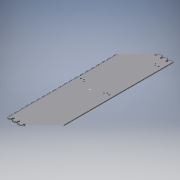
# Autodesk Inventor part: 3DPrinterBracket_bottom
Saved by Autodesk Inventor 2016 (Build 200138000, 138)
## iProperties
Created: 2017-10-03
Part Number: 3DPrinterBracket_bottom
Material: Generic
Document SubType Name: Modeling
Designer: jcj2131
Density: 1 g/cm^3
Appearance: Default
Author: jcj2131
Autodesk Inventor part; units mm, degrees
ref_plane "YZ Plane" through (0, 0, 0) normal (1, 0, 0) x (0, 1, 0)
ref_plane "XZ Plane" through (0, 0, 0) normal (0, 1, 0) x (-1, 0, 0)
ref_plane "XY Plane" through (0, 0, 0) normal (0, 0, 1) x (1, 0, 0)
sketch "Sketch1" plane through (0, 0, 0) normal (0, 1, 0) x (-1, 0, 0)
  line L0 (82.55, 306.3875) -> (-82.55, 306.3875)
  line L1 (-82.55, 306.3875) -> (-82.55, -306.3875)
  line L2 (-82.55, -306.3875) -> (82.55, -306.3875)
  line L3 (82.55, -306.3875) -> (82.55, 306.3875)
  point P0 (0, 0)
  point P1 (0, 306.3875)
  point P2 (82.55, 0)
  dimension "d0" = 612.775
  dimension "d1" = 165.1
  constraints: 8 end point, 2 midpoint, 2 parallel, 1 horizontal, 1 horizontal alignment, 1 perpendicular, 1 vertical alignment
  measures "d0" distance of L2.end L0.start
  measures "d1" distance of L0.start L0.end
extrude "Extrusion1" add sketch "Sketch1" along normal blind 3.175
sketch "Sketch2" plane through (0, 3.175, 0) normal (0, 1, 0) x (1, 0, 0)
  line L0 (-82.55, -306.3875) -> (82.55, -306.3875) projected
  line L1 (-69.85, -306.3875) -> (-57.15, -306.3875)
  line L2 (-57.15, -306.3875) -> (-57.15, -303.2125)
  line L3 (-57.15, -303.2125) -> (-69.85, -303.2125)
  line L4 (-69.85, -303.2125) -> (-69.85, -306.3875)
  line L5 (-82.55, 306.3875) -> (-82.55, -306.3875) projected
  point P0 (0, 0)
  dimension "d4" = 12.7
  dimension "d5" = 12.7
  dimension "d6" = 3.175
  constraints: 8 end point, 2 parallel, 1 horizontal, 1 perpendicular, 1 point on line
  measures "d4" distance between parallel lines of L5 L4
  measures "d5" distance of L2.end L3.end
  measures "d6" distance of L1.end L2.end
extrude "Extrusion2" cut sketch "Sketch2" against normal through all
sketch "Sketch3" plane through (0, 3.175, 0) normal (0, 1, 0) x (1, 0, 0)
  line L0 (-57.15, -303.2125) -> (-69.85, -303.2125) projected
  line L1 (-65.278, -303.2125) -> (-61.722, -303.2125)
  line L2 (-61.722, -303.2125) -> (-61.722, -297.2125)
  line L3 (-61.722, -297.2125) -> (-65.278, -297.2125)
  line L4 (-65.278, -297.2125) -> (-65.278, -303.2125)
  line L5 (-69.85, -306.3875) -> (-69.85, -303.2125) projected
  point P0 (0, 0)
  dimension "d9" = 3.556
  dimension "d10" = 6
  dimension "d11" = 4.572
  constraints: 8 end point, 2 parallel, 1 horizontal, 1 perpendicular, 1 point on line
  measures "d9" distance of L2.end L3.end
  measures "d10" distance of L3.end L1.start
  measures "d11" distance between parallel lines of L5 L4
extrude "Extrusion3" cut sketch "Sketch3" against normal through all
sketch "Sketch4" plane through (0, 3.175, 0) normal (0, 1, 0) x (1, 0, 0)
  line L0 (-59.5315, -297.2125) -> (-67.469, -297.2125)
  line L1 (-67.469, -297.2125) -> (-67.469, -294.4345)
  line L2 (-67.469, -294.4345) -> (-59.5315, -294.4345)
  line L3 (-59.5315, -294.4345) -> (-59.5315, -297.2125)
  line L4 (-65.278, -297.2125) -> (-61.722, -297.2125) projected
  line L5 (-69.85, -306.3875) -> (-69.85, -303.2125) projected
  point P0 (0, 0)
  dimension "d14" = 7.9375
  dimension "d15" = 2.778
  dimension "d16" = 0
  dimension "d17" = 2.381
  constraints: 8 end point, 2 parallel, 1 horizontal, 1 perpendicular
  measures "d14" distance of L1.end L2.end
  measures "d15" distance of L0.end L1.end
  measures "d16" distance between parallel lines of L4 L0
  measures "d17" distance between parallel lines of L5 L1
extrude "Extrusion4" cut sketch "Sketch4" against normal through all
sketch "Sketch5" plane through (0, 3.175, 0) normal (0, 1, 0) x (1, 0, 0)
  line L0 (-59.5315, -294.4345) -> (-67.469, -294.4345) projected
  line L1 (-65.278, -294.4345) -> (-61.722, -294.4345)
  line L2 (-61.722, -294.4345) -> (-61.722, -291.1475)
  line L3 (-61.722, -291.1475) -> (-65.278, -291.1475)
  line L4 (-65.278, -291.1475) -> (-65.278, -294.4345)
  line L5 (-69.85, -306.3875) -> (-69.85, -303.2125) projected
  line L6 (-57.15, -306.3875) -> (82.55, -306.3875) projected
  point P0 (0, 0)
  dimension "d20" = 3.556
  dimension "d21" = 4.572
  dimension "d22" = 15.24
  constraints: 8 end point, 2 parallel, 1 horizontal, 1 perpendicular, 1 point on line
  measures "d20" distance of L2.end L3.end
  measures "d21" distance between parallel lines of L5 L4
  measures "d22" distance between parallel lines of L6 L3
extrude "Extrusion5" cut sketch "Sketch5" against normal through all
pattern_linear "Rectangular Pattern1" count 6 spacing 25.4 along (1, 0, 0) of "Extrusion2", "Extrusion3", "Extrusion4", "Extrusion5"
sketch "Sketch6" plane through (0, 3.175, 0) normal (0, 1, 0) x (1, 0, 0)
  point P0 (0, 0)
mirror "Mirror1" about plane through (0, 0, 0) normal (0, 0, 1) of "Extrusion5", "Extrusion2", "Extrusion3", "Extrusion4", "Rectangular Pattern1"
sketch "Sketch7" plane through (0, 3.175, 0) normal (0, 1, 0) x (1, 0, 0)
  point P0 (0, 0)
sketch "Sketch8" plane through (0, 3.175, 0) normal (0, 1, 0) x (1, 0, 0)
  line L0 (-50.8, 22.3875) -> (50.8, 22.3875)
  line L1 (50.8, 22.3875) -> (50.8, 255.5875)
  line L2 (50.8, 255.5875) -> (-50.8, 255.5875)
  line L3 (-50.8, 255.5875) -> (-50.8, 22.3875)
  line L4 (-61.5, 148.8875) -> (61.5, 148.8875)
  line L5 (61.5, 148.8875) -> (61.5, 248.8875)
  line L6 (61.5, 248.8875) -> (-61.5, 248.8875)
  line L7 (-61.5, 248.8875) -> (-61.5, 148.8875)
  line L8 (82.55, -306.3875) -> (82.55, 306.3875) projected
  line L9 (-82.55, 306.3875) -> (-82.55, -306.3875) projected
  line L10 (-19.05, 306.3875) -> (-31.75, 306.3875) projected
  line L11 (-69.85, 306.3875) -> (-82.55, 306.3875) projected
  circle A0 centre (-57.5, 244.8875) radius 2.54
  circle A1 centre (-57.5, 152.8875) radius 2.54
  circle A2 centre (57.5, 152.8875) radius 2.54
  circle A3 centre (57.5, 244.8875) radius 2.54
  line L12 (-69.85, 306.3875) -> (-82.55, 306.3875) projected
  circle A4 centre (-54.61, 26.4875) radius 1.85
  circle A5 centre (-46.7, 18.5775) radius 1.85
  circle A6 centre (46.7, 18.5775) radius 1.85
  circle A7 centre (54.61, 26.4875) radius 1.85
  circle A8 centre (-54.61, 251.4875) radius 1.85
  circle A9 centre (-46.7, 259.3975) radius 1.85
  circle A10 centre (54.61, 251.4875) radius 1.85
  circle A11 centre (46.7, 259.3975) radius 1.85
  line L13 (-61.5, 128.8875) -> (61.5, 128.8875)
  line L14 (61.5, 128.8875) -> (61.5, 28.8875)
  line L15 (61.5, 28.8875) -> (-61.5, 28.8875)
  line L16 (-61.5, 28.8875) -> (-61.5, 128.8875)
  line L17 (-71.5, 258.8875) -> (-26.5, 258.8875)
  line L18 (-26.5, 258.8875) -> (-26.5, 18.8875)
  line L19 (-26.5, 18.8875) -> (-71.5, 18.8875)
  line L20 (-71.5, 18.8875) -> (-71.5, 258.8875)
  circle A12 centre (-66.5, 253.8875) radius 2.5
  circle A13 centre (-66.5, 23.8875) radius 2.5
  line L21 (26.5, 258.8875) -> (71.5, 258.8875)
  line L22 (71.5, 258.8875) -> (71.5, 18.8875)
  line L23 (71.5, 18.8875) -> (26.5, 18.8875)
  line L24 (26.5, 18.8875) -> (26.5, 258.8875)
  circle A14 centre (66.5, 253.8875) radius 2.5
  circle A15 centre (66.5, 23.8875) radius 2.5
  point P0 (0, 0)
  dimension "d28" = 233.2
  dimension "d29" = 101.6
  dimension "d30" = 100
  dimension "d31" = 123
  dimension "d36" = 5.08
  dimension "d37" = 4
  dimension "d38" = 4
  dimension "d39" = 5.08
  dimension "d40" = 4
  dimension "d41" = 4
  dimension "d42" = 5.08
  dimension "d43" = 4
  dimension "d44" = 4
  dimension "d45" = 5.08
  dimension "d46" = 4
  dimension "d47" = 4
  dimension "d73" = 21.05
  dimension "d74" = 10.7
  dimension "d75" = 50.8
  dimension "d76" = 57.5
  dimension "d77" = 3.7
  dimension "d78" = 3.81
  dimension "d79" = 4.1
  dimension "d80" = 3.7
  dimension "d81" = 3.81
  dimension "d82" = 4.1
  dimension "d83" = 3.7
  dimension "d84" = 3.81
  dimension "d85" = 4.1
  dimension "d86" = 3.7
  dimension "d87" = 3.81
  dimension "d88" = 3.7
  dimension "d89" = 3.81
  dimension "d90" = 4.1
  dimension "d91" = 3.7
  dimension "d92" = 3.81
  dimension "d93" = 4.1
  dimension "d94" = 3.7
  dimension "d95" = 3.81
  dimension "d96" = 4.1
  dimension "d97" = 3.7
  dimension "d98" = 3.81
  dimension "d99" = 4.1
  dimension "d109" = 4.1
  dimension "d118" = 20
  dimension "d119" = 240
  dimension "d120" = 45
  dimension "d121" = 14
  dimension "d122" = 14
  dimension "d123" = 5
  dimension "d124" = 5
  dimension "d125" = 5
  dimension "d126" = 5
  dimension "d127" = 5
  dimension "d128" = 5
  dimension "d129" = 53
  dimension "d130" = 5
  dimension "d131" = 5
  dimension "d132" = 5
  dimension "d133" = 14
  dimension "d134" = 5
  dimension "d135" = 5
  dimension "d136" = 5
  constraints: 40 end point, 16 centre point, 10 parallel, 5 horizontal, 5 perpendicular, 4 equal length
  measures "d28" distance of L2.end L0.start
  measures "d29" distance of L0.start L0.end
  measures "d30" distance of L6.end L4.start
  measures "d31" distance of L5.end L6.end
  measures "d36" diameter of A0
  measures "d37" distance from line of L6 A0.centre
  measures "d38" distance from line of L7 A0.centre
  measures "d39" diameter of A1
  measures "d40" distance from line of L7 A1.centre
  measures "d41" distance from line of L4 A1.centre
  measures "d42" diameter of A2
  measures "d43" distance from line of L5 A2.centre
  measures "d44" distance from line of L4 A2.centre
  measures "d45" diameter of A3
  measures "d46" distance from line of L5 A3.centre
  measures "d47" distance from line of L6 A3.centre
  measures "d73" distance between parallel lines of L8 L5
  measures "d74" distance between parallel lines of L5 L1
  measures "d75" distance between parallel lines of L11 L2
  measures "d76" distance between parallel lines of L12 L6
  measures "d77" diameter of A4
  measures "d78" distance from line of L3 A4.centre
  measures "d79" distance from line of L0 A4.centre
  measures "d80" diameter of A5
  measures "d81" distance from line of L0 A5.centre
  measures "d82" distance from line of L3 A5.centre
  measures "d83" diameter of A6
  measures "d84" distance from line of L0 A6.centre
  measures "d85" distance from line of L1 A6.centre
  measures "d86" diameter of A7
  measures "d87" distance from line of L1 A7.centre
  measures "d88" diameter of A8
  measures "d89" distance from line of L3 A8.centre
  measures "d90" distance from line of L2 A8.centre
  measures "d91" diameter of A9
  measures "d92" distance from line of L2 A9.centre
  measures "d93" distance from line of L3 A9.centre
  measures "d94" diameter of A10
  measures "d95" distance from line of L1 A10.centre
  measures "d96" distance from line of L2 A10.centre
  measures "d97" diameter of A11
  measures "d98" distance from line of L2 A11.centre
  measures "d99" distance from line of L1 A11.centre
  measures "d109" distance from line of L0 A7.centre
  measures "d118" distance between parallel lines of L13 L4
  measures "d119" distance of L19.end L17.start
  measures "d120" distance of L17.start L17.end
  measures "d121" distance from line of L20 A0.centre
  measures "d122" distance from line of A0.centre L17
  measures "d123" diameter of A12
  measures "d124" distance from line of L17 A12.centre
  measures "d125" distance from line of L20 A12.centre
  measures "d126" diameter of A13
  measures "d127" distance from line of L20 A13.centre
  measures "d128" distance from line of L19 A13.centre
  measures "d129" distance between parallel lines of L18 L24
  measures "d130" diameter of A14
  measures "d131" distance from line of L21 A14.centre
  measures "d132" distance from line of L22 A14.centre
  measures "d133" distance from line of L21 A3.centre
  measures "d134" diameter of A15
  measures "d135" distance from line of L22 A15.centre
  measures "d136" distance from line of L23 A15.centre
sketch "Sketch12" plane through (0, 3.175, 0) normal (0, 1, 0) x (1, 0, 0)
  line L0 (-82.55, -306.3875) -> (-79.375, -306.3875)
  line L1 (-79.375, -306.3875) -> (-79.375, -293.6875)
  line L2 (-79.375, -293.6875) -> (-82.55, -293.6875)
  line L3 (-82.55, -293.6875) -> (-82.55, -306.3875)
  line L4 (-82.55, -306.3875) -> (-69.85, -306.3875) projected
  line L5 (-82.55, 306.3875) -> (-82.55, -306.3875) projected
  point P0 (0, 0)
  dimension "d55" = 3.175
  dimension "d56" = 12.7
  dimension "d57" = 0
  dimension "d110" = 0
  constraints: 8 end point, 2 parallel, 1 horizontal, 1 perpendicular
  measures "d55" distance of L1.end L2.end
  measures "d56" distance of L0.end L1.end
  measures "d57" distance between parallel lines of L4 L0
  measures "d110" distance between parallel lines of L5 L3
extrude "Extrusion6" cut sketch "Sketch12" against normal through all
sketch "Sketch13" plane through (0, 3.175, 0) normal (0, 1, 0) x (1, 0, 0)
  line L0 (-82.55, -289.0901) -> (-79.375, -289.0901)
  line L1 (-79.375, -289.0901) -> (-79.375, -285.5341)
  line L2 (-79.375, -285.5341) -> (-82.55, -285.5341)
  line L3 (-82.55, -285.5341) -> (-82.55, -289.0901)
  line L4 (-82.55, -293.6875) -> (-79.375, -293.6875) projected
  line L5 (-82.55, 306.3875) -> (-82.55, -293.6875) projected
  point P0 (0, 0)
  dimension "d60" = 3.175
  dimension "d61" = 3.556
  dimension "d62" = 4.5974
  dimension "d111" = 0
  constraints: 8 end point, 2 parallel, 1 horizontal, 1 perpendicular
  measures "d60" distance of L1.end L2.end
  measures "d61" distance of L0.end L1.end
  measures "d62" distance between parallel lines of L4 L0
  measures "d111" distance between parallel lines of L5 L3
extrude "Extrusion7" cut sketch "Sketch13" against normal through all
pattern_linear "Rectangular Pattern2" count 23 spacing 25.4 along (0, 0, -1) of "Extrusion6", "Extrusion7"
extrude "Extrusion9" cut sketch "Sketch8" against normal through all contours L19 A5 | A5 L19 | L23 A6 | A6 L23 | L17 A9 | A9 L17 | L21 A11 | A11 L21 | A4 | A7 | A8 | A10
sketch "Sketch16" plane through (0, 3.175, 0) normal (0, 1, 0) x (1, 0, 0)
  line L0 (-82.55, 306.3875) -> (-82.55, 273.2659) projected
  line L1 (-82.55, 306.3875) -> (-79.375, 306.3875)
  line L2 (-79.375, 306.3875) -> (-79.375, 277.7875)
  line L3 (-79.375, 277.7875) -> (-82.55, 277.7875)
  line L4 (-82.55, 277.7875) -> (-82.55, 306.3875)
  line L5 (-82.55, 273.2659) -> (-79.375, 273.2659) projected
  point P0 (0, 0)
  dimension "d112" = 3.175
  dimension "d139" = 28.6
  constraints: 8 end point, 2 parallel, 1 horizontal, 1 perpendicular
  measures "d112" distance of L2.end L3.end
  measures "d139" distance of L1.end L2.end
extrude "Extrusion10" cut sketch "Sketch16" against normal through all
extrude "Extrusion12" cut sketch "Sketch8" against normal through all contours A12 | A13 | A14 | A15
equation "\"d58\" = d47"
equation "\"d63\" = d47"
body "Solid1"
